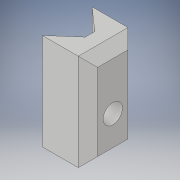
# Autodesk Inventor part: nut_part
Saved by Autodesk Inventor 2019 (Build 230136000, 136)
## iProperties
Created: 2021-10-21
Part Number: nut_part
Material: Genérico
Document SubType Name: Modeling
Designer: Juan M. Casillas
Density: 1 g/cm^3
Appearance: Valor por defecto
Author: Juan M. Casillas
Autodesk Inventor part; units mm, degrees
ref_plane "YZ Plane" through (0, 0, 0) normal (1, 0, 0) x (0, 1, 0)
ref_plane "XZ Plane" through (0, 0, 0) normal (0, 1, 0) x (-1, 0, 0)
ref_plane "XY Plane" through (0, 0, 0) normal (0, 0, 1) x (1, 0, 0)
sketch "Sketch1" plane through (0, 0, 0) normal (0, 1, 0) x (-1, 0, 0)
  line L0 (4.725, 5.15) -> (-4.725, 5.15)
  line L1 (-4.725, 5.15) -> (-4.725, -5.15)
  line L2 (-4.725, -5.15) -> (4.725, -5.15)
  line L3 (4.725, 5.15) -> (-4.725, -5.15) construction
  line L4 (-4.725, 5.15) -> (4.725, -5.15) construction
  line L5 (0, 0) -> (0, -1)
  line L6 (0, 0) -> (0, 1)
  line L7 (0, -1) -> (4.725, -5.15)
  line L8 (0, 1) -> (4.725, 5.15)
  dimension "d0" = 9.45
  dimension "d1" = 10.3
  dimension "d2" = 1
  dimension "d3" = 1
  constraints: 18 end point, 2 midpoint, 1 horizontal, 1 parallel, 1 perpendicular, 1 point on line, 1 vertical
  measures "d0" distance of L2.end L1.end
  measures "d1" distance of L1.end L0.end
  measures "d2" distance of L5.start L5.end
  measures "d3" distance of L5.start L6.end
extrude "Extrusion1" add sketch "Sketch1" along normal blind 20
sketch "Sketch2" plane through (4.725, 0, 5.15) normal (1, 0, 0) x (0, 0, -1)
  line L0 (10.3, 0) -> (0, 0) construction
  line L1 (10.3, 0) -> (10.3, 20) construction
  line L2 (0, 20) -> (10.3, 20) construction
  line L3 (0, 0) -> (0, 20) construction
  point P0 (5.15, 0)
  point P1 (5.15, 8.125)
hole "Hole1" at (4.725, 8.125, 0) direction (-1, 0, 0) diameter 4 end through all
chamfer "Chamfer1" distance 2 angle 45 4 edges at (4.725, 10, 5.15) (4.725, 0, 0) (4.725, 10, -5.15) (4.725, 20, 0)
body "Solid1"
